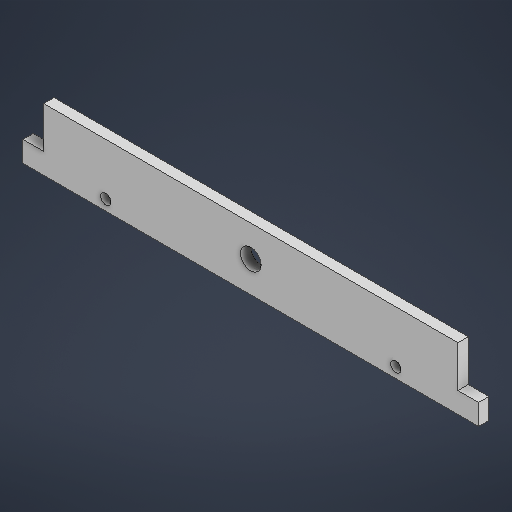
# Autodesk Inventor part: Part2
Saved by Autodesk Inventor 2026.1 (Build 301233020, 233B)
## iProperties
Created: 2025-11-02
Part Number: Part2
Material: Generic
Document SubType Name: Modeling
Designer: gusta
Density: 1 g/cm^3
Appearance: Default
Author: gusta
Autodesk Inventor part; units mm, degrees
ref_plane "YZ Plane" through (0, 0, 0) normal (1, 0, 0) x (0, 1, 0)
ref_plane "XZ Plane" through (0, 0, 0) normal (0, 1, 0) x (-1, 0, 0)
ref_plane "XY Plane" through (0, 0, 0) normal (0, 0, 1) x (1, 0, 0)
sketch "Sketch1" plane through (0, 0, 0) normal (0, 0, 1) x (1, 0, 0)
  line L0 (0, 0) -> (0, 20)
  line L1 (0, 20) -> (20, 20)
  line L2 (20, 20) -> (20, 60)
  line L3 (20, 60) -> (420, 60)
  line L4 (420, 60) -> (420, 20)
  line L5 (420, 20) -> (440, 20)
  line L6 (440, 20) -> (440, 0)
  line L7 (440, 0) -> (0, 0)
  dimension "d0" = 20
  dimension "d1" = 20
  dimension "d2" = 40
  dimension "d3" = 400
  dimension "d4" = 40
  dimension "d5" = 20
  constraints: 16 end point, 6 perpendicular, 2 vertical
  measures "d0" distance of L0.start L0.end
  measures "d1" distance of L0.end L1.end
  measures "d2" distance of L1.end L2.end
  measures "d3" distance of L2.end L3.end
  measures "d4" distance of L3.end L4.end
  measures "d5" distance of L4.end L5.end
extrude "Extrusion1" add sketch "Sketch1" along normal blind 10
sketch "Sketch2" plane through (0, 0, 10) normal (0, 0, 1) x (1, 0, 0)
  line L0 (20, 60) -> (20, 20) projected
  line L1 (0, 0) -> (440, 0) projected
  point P0 (80, 10)
  dimension "d8" = 60
  dimension "d16" = 10
  measures "d8" distance from line of L0 point (80, 10)
  measures "d16" distance from line of L1 point (80, 10)
hole "Hole1" at (80, 10, 10) direction (0, 0, -1) diameter 10 end through all
sketch "Sketch3" plane through (0, 0, 10) normal (0, 0, 1) x (1, 0, 0)
  line L0 (420, 20) -> (420, 60) projected
  line L1 (0, 0) -> (440, 0) projected
  point P0 (360, 10)
  dimension "d17" = 60
  dimension "d25" = 10
  measures "d17" distance from line of L0 point (360, 10)
  measures "d25" distance from line of L1 point (360, 10)
hole "Hole2" at (360, 10, 10) direction (0, 0, -1) diameter 10 end through all
sketch "Sketch4" plane through (0, 0, 10) normal (0, 0, 1) x (1, 0, 0)
  line L0 (20, 60) -> (20, 20) projected
  line L1 (0, 0) -> (440, 0) projected
  point P0 (220, 30)
  dimension "d26" = 200
  dimension "d34" = 30
  measures "d26" distance from line of L0 point (220, 30)
  measures "d34" distance from line of L1 point (220, 30)
hole "Hole3" at (220, 30, 10) direction (0, 0, -1) diameter 20 end through all
body "Solid1"
